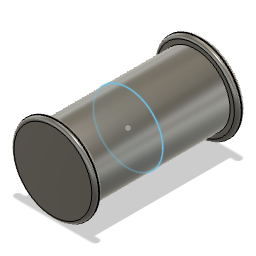
Lock slider and main base (Autodesk Fusion 360 design; units mm, degrees)
Autodesk Fusion 360 part; units mm, degrees
sketch "sketch 622" plane through (0, 0, 0) normal (0, 0, 1) x (1, 0, 0)
  circle A0 centre (14, -26.4187) radius 9
extrude "Extrude1" add sketch "sketch 622" along normal mid plane 35
sketch "Sketch1" plane through (0, 0, 17.5) normal (0, 0, 1) x (1, 0, 0)
  circle A0 centre (14, -26.4187) radius 9
  circle A1 centre (14, -26.4187) radius 11
  dimension "d68" = 22
  constraint concentric A0 A1
  measures "d68" diameter of A1
extrude "Extrude2" add sketch "Sketch1" along normal blind 2 contours A0 | A1
sketch "Sketch2" plane through (0, 0, -17.5) normal (0, 0, -1) x (-1, 0, 0)
  circle A0 centre (-14, -26.4187) radius 9
  circle A1 centre (-14, -26.4187) radius 11
  dimension "d71" = 22
  constraint concentric A0 A1
  measures "d71" diameter of A1
extrude "Extrude3" add sketch "Sketch2" along normal blind 2 contours A0 | A1
fillet "Fillet1" radius 0.9 2 edges at (3.7444, -30.3965, 17.5) (3.7444, -30.3965, 19.5)
fillet "Fillet2" radius 0.9 2 edges at (24.2556, -30.3965, -19.5) (24.2556, -30.3965, -17.5)
